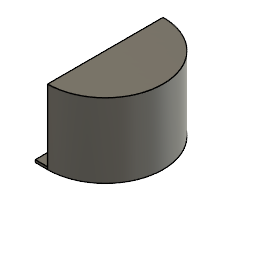
Connector Extension (Autodesk Fusion 360 design; units mm, degrees)
part number: 2026-06-01-17-57-32-068
Autodesk Fusion 360 part; units mm, degrees
sketch "Sketch1" plane through (0, 0, 0) normal (0, 1, 0) x (1, 0, 0)
  arc A0 (0, -23.375) -> (0, 23.375) centre (0, 0) ccw
  arc A1 (0, -23.375) -> (0, 23.375) centre (0, 0) ccw
  line L0 (0, -23.375) -> (0, 23.375)
  constraint coincident A0.end A1.end
  constraint coincident A0.start A1.start
  constraint vertical L0
  constraint coincident A0.centre A1.centre
  constraint vertical A0.start A0.centre
extrude "Extrude1" add sketch "Sketch1" along normal blind 30
sketch "Sketch2" plane through (0, 0, 0) normal (-1, 0, 0) x (0, 0, 1)
  line L0 (-23.375, 0) -> (23.375, 0)
  line L1 (23.375, 0) -> (23.375, 30)
  line L2 (23.375, 30) -> (-23.375, 30)
  line L3 (-23.375, 30) -> (-23.375, 0)
  line L4 (-23.375, 10) -> (0, 10)
  line L5 (0, 10) -> (0, -15)
  line L6 (0, -15) -> (-23.375, -15)
  line L7 (-23.375, -15) -> (-23.375, 10)
  constraint horizontal L4
  constraint vertical L5
  constraint horizontal L6
  constraint vertical L7
  constraint coincident L3 L4.start
extrude "Extrude2" add sketch "Sketch2" along normal blind 5 contours L0 L3 L4 L5 L7 | L0 L5 L6 L7
sketch "Sketch4" plane through (0, 0, 0) normal (0, 1, 0) x (1, 0, 0)
  line L0 (0, 0) -> (-5, 0)
  line L1 (-5, 0) -> (-5, -23.375)
  line L2 (-5, -23.375) -> (0, -23.375)
  line L3 (0, -23.375) -> (0, 0)
  point P0 (0, -23.375)
  constraint horizontal L0
  constraint vertical L1
  constraint horizontal L2
  constraint vertical L3
  constraint coincident L0.start L3.end
  constraint coincident P0 L2.end
extrude "Extrude3" add sketch "Sketch4" along normal blind 1
